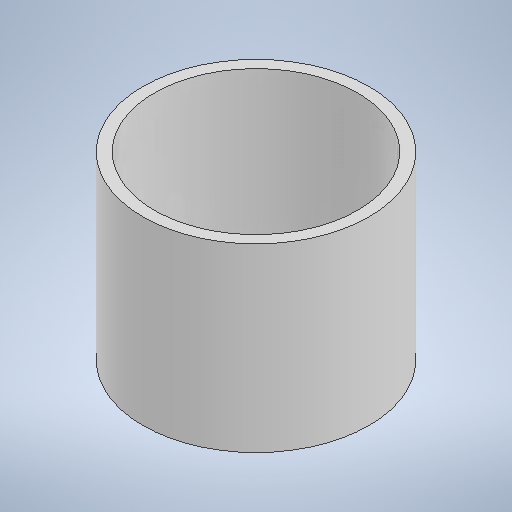
# Autodesk Inventor part: Walec
Saved by Autodesk Inventor 2025 (Build 290162000, 162)
## iProperties
Created: 2024-12-31
Part Number: Walec
Material: Ogólny
Document SubType Name: Modeling
Designer: Laptop
Density: 1 g/cm^3
Appearance: Domyślna
Author: Laptop
Autodesk Inventor part; units mm, degrees
ref_plane "YZ Plane" through (0, 0, 0) normal (1, 0, 0) x (0, 1, 0)
ref_plane "XZ Plane" through (0, 0, 0) normal (0, 1, 0) x (-1, 0, 0)
ref_plane "XY Plane" through (0, 0, 0) normal (0, 0, 1) x (1, 0, 0)
sketch "Szkic1" plane through (0, 0, 0) normal (0, 1, 0) x (-1, 0, 0)
  circle A0 centre (0, 0) radius 50
  dimension "d0" = 100
  constraints: 1 centre point, 1 coincident
  measures "d0" diameter of A0
extrude "Wyciągnięcie proste1" add sketch "Szkic1" along normal blind 80
sketch "Szkic2" plane through (0, 80, 0) normal (0, 1, 0) x (1, 0, 0)
  circle A0 centre (0, 0) radius 45
  dimension "d3" = 90
  constraints: 1 centre point, 1 coincident
  measures "d3" diameter of A0
extrude "Wyciągnięcie proste2" cut sketch "Szkic2" against normal blind 75
sketch "Szkic3" plane through (0, 5, 0) normal (0, 1, 0) x (1, 0, 0)
  point P0 (0, 0)
sketch "Szkic4" plane through (0, 5, 0) normal (0, 1, 0) x (1, 0, 0)
  circle A0 centre (0, 0) radius 22.5
  dimension "d6" = 45
  constraints: 1 centre point, 1 coincident
  measures "d6" diameter of A0
extrude "Wyciągnięcie proste3" cut sketch "Szkic4" against normal blind 75
sketch "Szkic9" plane through (0, 5, 0) normal (0, 1, 0) x (1, 0, 0)
  point P0 (0, 0)
